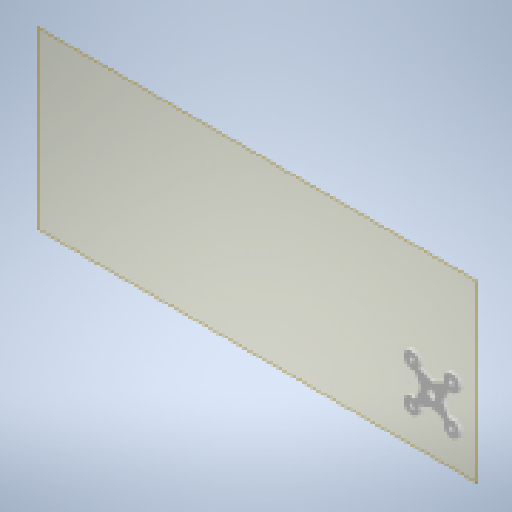
# Autodesk Inventor part: крепеж подшипника
Saved by Autodesk Inventor 2024.2 (Build 282272000, 272)
## iProperties
Created: 2026-02-22
Part Number: крепеж подшипника
Material: Типовые
Document SubType Name: Modeling
Designer: Service
Density: 1 g/cm^3
Appearance: По умолчанию
Author: Service
Autodesk Inventor part; units mm, degrees
ref_plane "YZ Plane" through (0, 0, 0) normal (1, 0, 0) x (0, 1, 0)
ref_plane "XZ Plane" through (0, 0, 0) normal (0, 1, 0) x (-1, 0, 0)
ref_plane "XY Plane" through (0, 0, 0) normal (0, 0, 1) x (1, 0, 0)
ref_plane "РабПлоскость1" through (-194.4569, -1.6478, -98.8355) normal (0, 0, 1) x (0, -1, 0)
sketch "Эскиз1" plane through (-194.4569, -1.6478, -98.8355) normal (0, 0, 1) x (0, -1, 0)
  circle A0 centre (5, 145) radius 1.5 projected
  circle A1 centre (5, 119) radius 1.5 projected
  circle A2 centre (18, 132) radius 7 projected
  circle A3 centre (31, 119) radius 1.5 projected
  circle A4 centre (31, 145) radius 1.5 projected
  line L0 (18.8381, 124.6132) -> (31, 119)
  line L1 (17.1619, 124.6132) -> (5, 119)
  line L2 (5, 119) -> (10.6132, 131.1619)
  line L3 (5, 145) -> (10.6132, 132.8381)
  line L4 (17.1619, 139.3868) -> (5, 145)
  line L5 (18.8381, 139.3868) -> (31, 145)
  line L6 (31, 145) -> (25.3868, 132.8381)
  line L7 (25.3868, 131.1619) -> (31, 119)
  circle A5 centre (5, 119) radius 5.275
  circle A6 centre (5, 145) radius 5.275
  circle A7 centre (31, 145) radius 5.275
  circle A8 centre (31, 119) radius 5.275
  arc A9 (18.8381, 124.6132) -> (17.1619, 124.6132) centre (18, 122.7973) ccw
  arc A10 (25.3868, 132.8381) -> (25.3868, 131.1619) centre (27.2027, 132) ccw
  arc A11 (17.1619, 139.3868) -> (18.8381, 139.3868) centre (18, 141.2027) ccw
  arc A12 (10.6132, 131.1619) -> (10.6132, 132.8381) centre (8.7973, 132) ccw
  circle A13 centre (18, 132) radius 2.75
  point P0 (-1.6478, 194.4569)
  point P1 (18, 125)
  point P2 (11, 132)
  point P3 (18, 139)
  point P4 (25, 132)
  point P5 (9.7895, 121.2105)
  point P6 (26.2105, 121.2105)
  point P7 (28.7895, 123.7895)
  point P8 (28.7895, 140.2105)
  point P9 (26.2105, 142.7895)
  point P10 (9.7895, 142.7895)
  point P11 (7.2105, 140.2105)
  point P12 (7.2105, 123.7895)
  point P13 (6.3619, 119.6286)
  point P14 (5.6286, 120.3619)
  point P15 (5.6286, 143.6381)
  point P16 (6.3619, 144.3714)
  point P17 (29.6381, 144.3714)
  point P18 (30.3714, 143.6381)
  point P19 (30.3714, 120.3619)
  point P20 (29.6381, 119.6286)
  dimension "d0" = 2
  dimension "d1" = 5.5
  constraints: 16 end point, 12 point on circle, 9 centre point, 8 point on line, 8 tangent, 5 coincident, 5 perpendicular, 3 equal radius
  measures "d0" radius of A9
  measures "d1" diameter of A13
extrude "Выдавливание1" add sketch "Эскиз1" along normal blind 2 contours A0 L3 A6 L4 | A0 L4 A6 L3 | A6 L4 A11 L5 A7 L6 A10 L7 A8 L0 A9 L1 A5 L2 A12 L3 | A5 L1 A1 L2 | L2 A1 L1 A5 | A7 L6 A4 L5 | L5 A4 L6 A7 | A8 L7 A3 L0 | L0 A3 L7 A8 | A2
